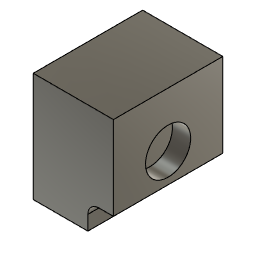
Grip Block v5 (Autodesk Fusion 360 design; units mm, degrees)
Autodesk Fusion 360 part; units mm, degrees
note: some values were not read from the file. Set by a fixed rule: which sketch regions a step uses.
sketch "Sketch1" plane through (0, 0, 0) normal (0, 0, 1) x (1, 0, 0)
  line L0 (0, 0) -> (22, 0)
  line L1 (22, 0) -> (22, 30)
  line L2 (22, 30) -> (0, 30)
  line L3 (0, 30) -> (0, 0)
  dimension "d3" = 22
  constraint horizontal L0
  constraint vertical L1
  constraint horizontal L2
  constraint vertical L3
  constraint coincident L0.start L3.end
  measures "d3" distance of L1 L3
extrude "Extrude1" add sketch "Sketch1" along normal blind 30
sketch "Sketch2" plane through (22, 0, 0) normal (1, 0, 0) x (0, 1, 0)
  line L0 (0, 0) -> (30, 0)
  line L1 (30, 0) -> (30, 30)
  line L2 (30, 30) -> (0, 30)
  line L3 (0, 30) -> (0, 0)
  circle A0 centre (15, 15) radius 6.2
  dimension "d4" = 12.4
  measures "d4" diameter of A0
extrude "Extrude2" cut sketch "Sketch2" against normal blind 5 contours A0
sketch "Sketch3" plane through (0, 0, 0) normal (0, -1, 0) x (1, 0, 0)
  line L0 (0, 0) -> (22, 0)
  line L1 (22, 0) -> (22, 30)
  line L2 (22, 30) -> (0, 30)
  line L3 (0, 30) -> (0, 0)
  circle A0 centre (18, 4) radius 2.5
  line L4 (22, 7) -> (18, 7)
  arc A1 (18, 7) -> (15, 4) centre (18, 4) ccw
  line L5 (15, 4) -> (15, 0)
  dimension "d7" = 5
  dimension "d8" = 4
  dimension "d9" = 4
  dimension "d13" = 7
  constraint coincident L1 L4.start
  constraint perpendicular L1 L4
  constraint tangent L4 A1
  constraint coincident L0 L5.end
  constraint tangent A1 L5
  measures "d7" diameter of A0
  measures "d8" distance of L1 A0.centre
  measures "d9" distance of L0 A0.centre
  measures "d13" distance of L0 L4
extrude "Extrude3" cut sketch "Sketch3" against normal blind 30 contours L0 L1 L4 A1 L5 | A0
